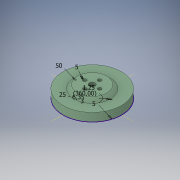
# Autodesk Inventor part: CircularSpline
Saved by Autodesk Inventor 2018.3 (Build 223284000, 284)
## iProperties
Created: 2018-06-23
Part Number: CircularSpline
Material: Generisch
Document SubType Name: Modeling
Designer: JochenAlt
Density: 1 g/cm^3
Appearance: Gummi - grün
Author: JochenAlt
Autodesk Inventor part; units mm, degrees
ref_plane "YZ Plane" through (0, 0, 0) normal (1, 0, 0) x (0, 1, 0)
ref_plane "XZ Plane" through (0, 0, 0) normal (0, 1, 0) x (-1, 0, 0)
ref_plane "XY Plane" through (0, 0, 0) normal (0, 0, 1) x (1, 0, 0)
sketch "Skizze1" plane through (0, 0, 0) normal (0, 0, 1) x (1, 0, 0)
  circle A0 centre (0, 0) radius 22.7501 construction
  circle A1 centre (0, 0) radius 20.6901 construction
  circle A2 centre (0, 0) radius 19.7501
  line L0 (0, 0) -> (5.4445, 22.0891) construction
  line L1 (0, 32.3027) -> (0, -32.3027) construction
  line L2 (-32.1257, 0) -> (32.1257, 0) construction
  arc A3 (1.4863, 21.1557) -> (0, 22.7501) centre (0, 21.2601) ccw
  line L3 (1.4863, 21.1557) -> (0, 0) construction
  line L4 (3.6197, 20.8967) -> (0, 0) construction
  line L5 (3.0398, 20.4656) -> (1.9462, 20.5984)
  arc A4 (1.4863, 21.1557) -> (1.9462, 20.5984) centre (2.0094, 21.119) ccw
  arc A5 (3.0398, 20.4656) -> (3.6197, 20.8967) centre (3.1031, 20.9862) ccw
  arc A6 (5.4445, 22.0891) -> (3.6197, 20.8967) centre (5.0879, 20.6424) ccw
  arc A7 (-3.6197, 20.8967) -> (-5.4445, 22.0891) centre (-5.0879, 20.6424) ccw
  arc A8 (-3.6197, 20.8967) -> (-3.0398, 20.4656) centre (-3.1031, 20.9862) ccw
  circle A9 centre (0, 0) radius 20.6901 construction
  line L6 (-1.9462, 20.5984) -> (-3.0398, 20.4656)
  arc A10 (-1.9462, 20.5984) -> (-1.4863, 21.1557) centre (-2.0094, 21.119) ccw
  arc A11 (0, 22.7501) -> (-1.4863, 21.1557) centre (0, 21.2601) ccw
  arc A12 (-8.5155, 19.4232) -> (-10.5725, 20.1443) centre (-9.8801, 18.8249) ccw
  arc A13 (-8.5155, 19.4232) -> (-7.8493, 19.1434) centre (-8.0352, 19.6337) ccw
  circle A14 centre (0, 0) radius 20.6901 construction
  line L7 (-6.8192, 19.5341) -> (-7.8493, 19.1434)
  arc A15 (-6.8192, 19.5341) -> (-6.506, 20.1853) centre (-7.0051, 20.0244) ccw
  arc A16 (-5.4445, 22.0891) -> (-6.506, 20.1853) centre (-5.0879, 20.6424) ccw
  arc A17 (-12.9163, 16.8209) -> (-15.0861, 17.0287) centre (-14.0981, 15.9134) ccw
  arc A18 (-12.9163, 16.8209) -> (-12.2025, 16.7087) centre (-12.5004, 17.1403) ccw
  circle A19 centre (0, 0) radius 20.6901 construction
  line L8 (-11.2959, 17.3345) -> (-12.2025, 16.7087)
  arc A20 (-11.2959, 17.3345) -> (-11.1476, 18.0417) centre (-11.5937, 17.7661) ccw
  arc A21 (-10.5725, 20.1443) -> (-11.1476, 18.0417) centre (-9.8801, 18.8249) ccw
  arc A22 (-16.5665, 13.241) -> (-18.723, 12.9236) centre (-17.4968, 12.0771) ccw
  arc A23 (-16.5665, 13.241) -> (-15.8466, 13.3029) centre (-16.2391, 13.6507) ccw
  circle A24 centre (0, 0) radius 20.6901 construction
  line L9 (-15.116, 14.1275) -> (-15.8466, 13.3029)
  arc A25 (-15.116, 14.1275) -> (-15.1414, 14.8497) centre (-15.5085, 14.4753) ccw
  arc A26 (-15.0861, 17.0287) -> (-15.1414, 14.8497) centre (-14.0981, 15.9134) ccw
  arc A27 (-19.2539, 8.8917) -> (-21.2718, 8.0673) centre (-19.8786, 7.539) ccw
  arc A28 (-19.2539, 8.8917) -> (-18.5697, 9.124) centre (-19.034, 9.3677) ccw
  circle A29 centre (0, 0) radius 20.6901 construction
  line L10 (-18.0577, 10.0995) -> (-18.5697, 9.124)
  arc A30 (-18.0577, 10.0995) -> (-18.2551, 10.7946) centre (-18.5221, 10.3432) ccw
  arc A31 (-18.723, 12.9236) -> (-18.2551, 10.7946) centre (-17.4968, 12.0771) ccw
  arc A32 (-20.8223, 4.0255) -> (-22.5843, 2.7422) centre (-21.1051, 2.5626) ccw
  arc A33 (-20.8223, 4.0255) -> (-20.2136, 4.4149) centre (-20.7228, 4.5404) ccw
  circle A34 centre (0, 0) radius 20.6901 construction
  line L11 (-19.95, 5.4845) -> (-20.2136, 4.4149)
  arc A35 (-19.95, 5.4845) -> (-20.308, 6.1122) centre (-20.4591, 5.61) ccw
  arc A36 (-21.2718, 8.0673) -> (-20.308, 6.1122) centre (-19.8786, 7.539) ccw
  arc A37 (-21.1806, -1.0745) -> (-22.5843, -2.7422) centre (-21.1051, -2.5626) ccw
  arc A38 (-21.1806, -1.0745) -> (-20.6828, -0.5508) centre (-21.2072, -0.5508) ccw
  circle A39 centre (0, 0) radius 20.6901 construction
  line L12 (-20.6828, 0.5508) -> (-20.6828, -0.5508)
  arc A40 (-20.6828, 0.5508) -> (-21.1806, 1.0745) centre (-21.2072, 0.5508) ccw
  arc A41 (-22.5843, 2.7422) -> (-21.1806, 1.0745) centre (-21.1051, 2.5626) ccw
  arc A42 (-20.308, -6.1122) -> (-21.2718, -8.0673) centre (-19.8786, -7.539) ccw
  arc A43 (-20.308, -6.1122) -> (-19.95, -5.4845) centre (-20.4591, -5.61) ccw
  circle A44 centre (0, 0) radius 20.6901 construction
  line L13 (-20.2136, -4.4149) -> (-19.95, -5.4845)
  arc A45 (-20.2136, -4.4149) -> (-20.8223, -4.0255) centre (-20.7228, -4.5404) ccw
  arc A46 (-22.5843, -2.7422) -> (-20.8223, -4.0255) centre (-21.1051, -2.5626) ccw
  arc A47 (-18.2551, -10.7946) -> (-18.723, -12.9236) centre (-17.4968, -12.0771) ccw
  arc A48 (-18.2551, -10.7946) -> (-18.0577, -10.0995) centre (-18.5221, -10.3432) ccw
  circle A49 centre (0, 0) radius 20.6901 construction
  line L14 (-18.5697, -9.124) -> (-18.0577, -10.0995)
  arc A50 (-18.5697, -9.124) -> (-19.2539, -8.8917) centre (-19.034, -9.3677) ccw
  arc A51 (-21.2718, -8.0673) -> (-19.2539, -8.8917) centre (-19.8786, -7.539) ccw
  arc A52 (-15.1414, -14.8497) -> (-15.0861, -17.0287) centre (-14.0981, -15.9134) ccw
  arc A53 (-15.1414, -14.8497) -> (-15.116, -14.1275) centre (-15.5085, -14.4753) ccw
  circle A54 centre (0, 0) radius 20.6901 construction
  line L15 (-15.8466, -13.3029) -> (-15.116, -14.1275)
  arc A55 (-15.8466, -13.3029) -> (-16.5665, -13.241) centre (-16.2391, -13.6507) ccw
  arc A56 (-18.723, -12.9236) -> (-16.5665, -13.241) centre (-17.4968, -12.0771) ccw
  arc A57 (-11.1476, -18.0417) -> (-10.5725, -20.1443) centre (-9.8801, -18.8249) ccw
  arc A58 (-11.1476, -18.0417) -> (-11.2959, -17.3345) centre (-11.5937, -17.7661) ccw
  circle A59 centre (0, 0) radius 20.6901 construction
  line L16 (-12.2025, -16.7087) -> (-11.2959, -17.3345)
  arc A60 (-12.2025, -16.7087) -> (-12.9163, -16.8209) centre (-12.5004, -17.1403) ccw
  arc A61 (-15.0861, -17.0287) -> (-12.9163, -16.8209) centre (-14.0981, -15.9134) ccw
  arc A62 (-6.506, -20.1853) -> (-5.4445, -22.0891) centre (-5.0879, -20.6424) ccw
  arc A63 (-6.506, -20.1853) -> (-6.8192, -19.5341) centre (-7.0051, -20.0244) ccw
  circle A64 centre (0, 0) radius 20.6901 construction
  line L17 (-7.8493, -19.1434) -> (-6.8192, -19.5341)
  arc A65 (-7.8493, -19.1434) -> (-8.5155, -19.4232) centre (-8.0352, -19.6337) ccw
  arc A66 (-10.5725, -20.1443) -> (-8.5155, -19.4232) centre (-9.8801, -18.8249) ccw
  arc A67 (-1.4863, -21.1557) -> (0, -22.7501) centre (0, -21.2601) ccw
  arc A68 (-1.4863, -21.1557) -> (-1.9462, -20.5984) centre (-2.0094, -21.119) ccw
  circle A69 centre (0, 0) radius 20.6901 construction
  line L18 (-3.0398, -20.4656) -> (-1.9462, -20.5984)
  arc A70 (-3.0398, -20.4656) -> (-3.6197, -20.8967) centre (-3.1031, -20.9862) ccw
  arc A71 (-5.4445, -22.0891) -> (-3.6197, -20.8967) centre (-5.0879, -20.6424) ccw
  arc A72 (3.6197, -20.8967) -> (5.4445, -22.0891) centre (5.0879, -20.6424) ccw
  arc A73 (3.6197, -20.8967) -> (3.0398, -20.4656) centre (3.1031, -20.9862) ccw
  circle A74 centre (0, 0) radius 20.6901 construction
  line L19 (1.9462, -20.5984) -> (3.0398, -20.4656)
  arc A75 (1.9462, -20.5984) -> (1.4863, -21.1557) centre (2.0094, -21.119) ccw
  arc A76 (0, -22.7501) -> (1.4863, -21.1557) centre (0, -21.2601) ccw
  arc A77 (8.5155, -19.4232) -> (10.5725, -20.1443) centre (9.8801, -18.8249) ccw
  arc A78 (8.5155, -19.4232) -> (7.8493, -19.1434) centre (8.0352, -19.6337) ccw
  circle A79 centre (0, 0) radius 20.6901 construction
  line L20 (6.8192, -19.5341) -> (7.8493, -19.1434)
  arc A80 (6.8192, -19.5341) -> (6.506, -20.1853) centre (7.0051, -20.0244) ccw
  arc A81 (5.4445, -22.0891) -> (6.506, -20.1853) centre (5.0879, -20.6424) ccw
  arc A82 (12.9163, -16.8209) -> (15.0861, -17.0287) centre (14.0981, -15.9134) ccw
  arc A83 (12.9163, -16.8209) -> (12.2025, -16.7087) centre (12.5004, -17.1403) ccw
  circle A84 centre (0, 0) radius 20.6901 construction
  line L21 (11.2959, -17.3345) -> (12.2025, -16.7087)
  arc A85 (11.2959, -17.3345) -> (11.1476, -18.0417) centre (11.5937, -17.7661) ccw
  arc A86 (10.5725, -20.1443) -> (11.1476, -18.0417) centre (9.8801, -18.8249) ccw
  arc A87 (16.5665, -13.241) -> (18.723, -12.9236) centre (17.4968, -12.0771) ccw
  arc A88 (16.5665, -13.241) -> (15.8466, -13.3029) centre (16.2391, -13.6507) ccw
  circle A89 centre (0, 0) radius 20.6901 construction
  line L22 (15.116, -14.1275) -> (15.8466, -13.3029)
  arc A90 (15.116, -14.1275) -> (15.1414, -14.8497) centre (15.5085, -14.4753) ccw
  arc A91 (15.0861, -17.0287) -> (15.1414, -14.8497) centre (14.0981, -15.9134) ccw
  arc A92 (19.2539, -8.8917) -> (21.2718, -8.0673) centre (19.8786, -7.539) ccw
  arc A93 (19.2539, -8.8917) -> (18.5697, -9.124) centre (19.034, -9.3677) ccw
  circle A94 centre (0, 0) radius 20.6901 construction
  line L23 (18.0577, -10.0995) -> (18.5697, -9.124)
  arc A95 (18.0577, -10.0995) -> (18.2551, -10.7946) centre (18.5221, -10.3432) ccw
  arc A96 (18.723, -12.9236) -> (18.2551, -10.7946) centre (17.4968, -12.0771) ccw
  arc A97 (20.8223, -4.0255) -> (22.5843, -2.7422) centre (21.1051, -2.5626) ccw
  arc A98 (20.8223, -4.0255) -> (20.2136, -4.4149) centre (20.7228, -4.5404) ccw
  circle A99 centre (0, 0) radius 20.6901 construction
  line L24 (19.95, -5.4845) -> (20.2136, -4.4149)
  arc A100 (19.95, -5.4845) -> (20.308, -6.1122) centre (20.4591, -5.61) ccw
  arc A101 (21.2718, -8.0673) -> (20.308, -6.1122) centre (19.8786, -7.539) ccw
  arc A102 (21.1806, 1.0745) -> (22.5843, 2.7422) centre (21.1051, 2.5626) ccw
  arc A103 (21.1806, 1.0745) -> (20.6828, 0.5508) centre (21.2072, 0.5508) ccw
  circle A104 centre (0, 0) radius 20.6901 construction
  line L25 (20.6828, -0.5508) -> (20.6828, 0.5508)
  arc A105 (20.6828, -0.5508) -> (21.1806, -1.0745) centre (21.2072, -0.5508) ccw
  arc A106 (22.5843, -2.7422) -> (21.1806, -1.0745) centre (21.1051, -2.5626) ccw
  arc A107 (20.308, 6.1122) -> (21.2718, 8.0673) centre (19.8786, 7.539) ccw
  arc A108 (20.308, 6.1122) -> (19.95, 5.4845) centre (20.4591, 5.61) ccw
  circle A109 centre (0, 0) radius 20.6901 construction
  line L26 (20.2136, 4.4149) -> (19.95, 5.4845)
  arc A110 (20.2136, 4.4149) -> (20.8223, 4.0255) centre (20.7228, 4.5404) ccw
  arc A111 (22.5843, 2.7422) -> (20.8223, 4.0255) centre (21.1051, 2.5626) ccw
  arc A112 (18.2551, 10.7946) -> (18.723, 12.9236) centre (17.4968, 12.0771) ccw
  arc A113 (18.2551, 10.7946) -> (18.0577, 10.0995) centre (18.5221, 10.3432) ccw
  circle A114 centre (0, 0) radius 20.6901 construction
  line L27 (18.5697, 9.124) -> (18.0577, 10.0995)
  arc A115 (18.5697, 9.124) -> (19.2539, 8.8917) centre (19.034, 9.3677) ccw
  arc A116 (21.2718, 8.0673) -> (19.2539, 8.8917) centre (19.8786, 7.539) ccw
  arc A117 (15.1414, 14.8497) -> (15.0861, 17.0287) centre (14.0981, 15.9134) ccw
  arc A118 (15.1414, 14.8497) -> (15.116, 14.1275) centre (15.5085, 14.4753) ccw
  circle A119 centre (0, 0) radius 20.6901 construction
  line L28 (15.8466, 13.3029) -> (15.116, 14.1275)
  arc A120 (15.8466, 13.3029) -> (16.5665, 13.241) centre (16.2391, 13.6507) ccw
  arc A121 (18.723, 12.9236) -> (16.5665, 13.241) centre (17.4968, 12.0771) ccw
  arc A122 (11.1476, 18.0417) -> (10.5725, 20.1443) centre (9.8801, 18.8249) ccw
  arc A123 (11.1476, 18.0417) -> (11.2959, 17.3345) centre (11.5937, 17.7661) ccw
  circle A124 centre (0, 0) radius 20.6901 construction
  line L29 (12.2025, 16.7087) -> (11.2959, 17.3345)
  arc A125 (12.2025, 16.7087) -> (12.9163, 16.8209) centre (12.5004, 17.1403) ccw
  arc A126 (15.0861, 17.0287) -> (12.9163, 16.8209) centre (14.0981, 15.9134) ccw
  arc A127 (6.506, 20.1853) -> (5.4445, 22.0891) centre (5.0879, 20.6424) ccw
  arc A128 (6.506, 20.1853) -> (6.8192, 19.5341) centre (7.0051, 20.0244) ccw
  circle A129 centre (0, 0) radius 20.6901 construction
  line L30 (7.8493, 19.1434) -> (6.8192, 19.5341)
  arc A130 (7.8493, 19.1434) -> (8.5155, 19.4232) centre (8.0352, 19.6337) ccw
  arc A131 (10.5725, 20.1443) -> (8.5155, 19.4232) centre (9.8801, 18.8249) ccw
  dimension "d0" = 3
  dimension "d1" = 2.06
  dimension "d2" = 13.846
  dimension "d3" = 41.3803
  dimension "d4" = 2.98
  dimension "d21" = 41.3803
  constraints: 288 point on circle, 132 centre point, 58 end point, 6 tangent, 3 coincident, 3 point on line
  measures "d0" radial gap between concentric circles of A0 A2
  measures "d1" radial gap between concentric circles of A0 A1
  measures "d2" angle of L0 L1
  measures "d3" diameter of A1
  measures "d4" diameter of A3
  measures "d21" diameter of A14
sketch "Skizze2" plane through (0, 0, 0) normal (0, 0, 1) x (1, 0, 0)
  circle A0 centre (0, 0) radius 20
  circle A1 centre (0, 0) radius 2.5
  circle A2 centre (0, 0) radius 25
  line L0 (0, 35) -> (0, -35) construction
  line L1 (-35, 0) -> (35, 0) construction
  circle A3 centre (-6.35, 0) radius 1.5
  circle A4 centre (0, 0) radius 12.5
  circle A5 centre (-6.35, 0) radius 2.75
  circle A6 centre (0, -6.35) radius 2.75
  circle A7 centre (0, -6.35) radius 1.5
  circle A8 centre (6.35, 0) radius 2.75
  circle A9 centre (6.35, 0) radius 1.5
  circle A10 centre (0, 6.35) radius 2.75
  circle A11 centre (0, 6.35) radius 1.5
  dimension "d15" = 5
  dimension "d22" = 5
  dimension "d23" = 50
  dimension "d25" = 3
  dimension "d26" = 6.35
  dimension "d31" = 25
  dimension "d35" = 1.25
  dimension "d38" = 360
  constraints: 12 centre point, 8 coincident, 1 point on line, 17 other
  measures "d15" diameter of A1
  measures "d22" radial gap between concentric circles of A2 A0
  measures "d23" diameter of A2
  measures "d25" diameter of A3
  measures "d26" distance of A3.centre point (0, 0)
  measures "d31" diameter of A4
  measures "d35" radial gap between concentric circles of A5 A3
extrude "Extrusion1" add sketch "Skizze2" along normal blind 7 contours A0 | A2 | A4
extrude "Extrusion2" cut sketch "Skizze1" along normal blind 4 contours A2 | A4 L5 A5 A6 A127 A128 L30 A130 A131 A122 A123 L29 A125 A126 A117 A118 L28 A120 A121 A112 A113 L27 A115 A116 A107 A108 L26 A110 A111 A102 A103 L25 A105 A106 A97 A98 L24 A100 A101 A92 A93 L23 A95 A96 A87 A88 L22 A90 A91 A82 A83 L21 A85 A86 A77 A78 L20 A80 A81 A72 A73 L19 A75 A76 A67 A68 L18 A70 A71 A62 A63 L17 A65 A66 A57 A58 L16 A60 A61 A52 A53 L15 A55 A56 A47 A48 L14 A50 A51 A42 A43 L13 A45 A46 A37 A38 L12 A40 A41 A32 A33 L11 A35 A36 A27 A28 L10 A30 A31 A22 A23 L9 A25 A26 A17 A18 L8 A20 A21 A12 A13 L7 A15 A16 A7 A8 L6 A10 A11 A3
extrude "Extrusion3" add sketch "Skizze2" along normal blind 3 from surface at 7 contours A4 | A5 | A6 | A8 | A10
chamfer "Fase1" distance 3 angle 45 1 edges at (-12.5, 0, 7)
